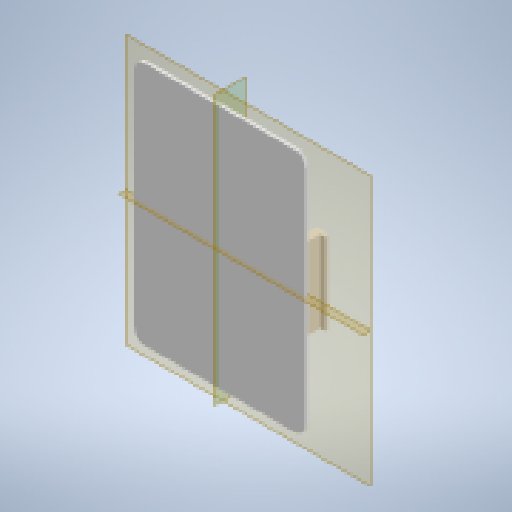
# Autodesk Inventor part: lidV2
Saved by Autodesk Inventor 2025.2 (Build 292293000, 293)
## iProperties
Created: 2022-04-11
Part Number: lidV2
Material: Generic
Document SubType Name: Modeling
Designer: Fred
Density: 1 g/cm^3
Appearance: Default
Author: Fred
Autodesk Inventor part; units mm, degrees
ref_plane "YZ Plane" through (0, 0, 0) normal (1, 0, 0) x (0, 1, 0)
ref_plane "XZ Plane" through (0, 0, 0) normal (0, 1, 0) x (-1, 0, 0)
ref_plane "XY Plane" through (0, 0, 0) normal (0, 0, 1) x (1, 0, 0)
ref_plane "Work Plane1" through (0, 0, 0) normal (0, 0, 1) x (1, 0, 0)
sketch "Sketch1" plane through (0, 0, 0) normal (0, 0, 1) x (1, 0, 0)
  arc A0 (14.605, -35.56) -> (17.78, -32.385) centre (14.605, -32.385) ccw projected
  line L0 (17.78, -32.385) -> (17.78, 33.985) projected
  arc A1 (17.78, 33.985) -> (14.605, 37.16) centre (14.605, 33.985) ccw projected
  line L1 (14.605, 37.16) -> (-29.845, 37.16) projected
  arc A2 (-29.845, 37.16) -> (-33.02, 33.985) centre (-29.845, 33.985) ccw projected
  line L2 (-33.02, 33.985) -> (-33.02, -32.385) projected
  arc A3 (-33.02, -32.385) -> (-29.845, -35.56) centre (-29.845, -32.385) ccw projected
  line L3 (-29.845, -35.56) -> (14.605, -35.56) projected
  line L4 (13.105, -34.06) -> (-28.345, -34.06) projected
  arc A4 (-31.52, -30.885) -> (-28.345, -34.06) centre (-28.345, -30.885) ccw projected
  line L5 (-31.52, -30.885) -> (-31.52, 30.885) projected
  arc A5 (-28.345, 34.06) -> (-31.52, 30.885) centre (-28.345, 30.885) ccw projected
  line L6 (-28.345, 34.06) -> (13.105, 34.06) projected
  arc A6 (16.28, 30.885) -> (13.105, 34.06) centre (13.105, 30.885) ccw projected
  line L7 (16.28, 30.885) -> (16.28, -30.885) projected
  arc A7 (13.105, -34.06) -> (16.28, -30.885) centre (13.105, -30.885) ccw projected
  point P0 (0, 0)
extrude "Extrusion1" add sketch "Sketch1" along normal blind 1 contours L3 A3 L2 A2 L1 A1 L0 A0 | L4 A4 L5 A5 L6 A6 L7 A7
ref_plane "Work Plane2" through (-29.845, 0.8, 0) normal (0, 1, 0) x (1, 0, 0)
sketch "Sketch3" plane through (-29.845, 0.8, 0) normal (0, 1, 0) x (1, 0, 0)
  line L0 (46.125, 31.5) -> (46.125, 0) projected
  line L1 (47.625, 5) -> (47.625, 7) projected
  line L2 (46.125, 5) -> (47.625, 5) projected
  line L3 (46.125, 7) -> (46.125, 5) projected
  line L4 (46.125, 7) -> (47.625, 7) projected
  line L5 (43.375, 0) -> (43.375, 6.8424)
  line L6 (43.375, 6.8424) -> (45.775, 6.8424)
  line L7 (45.775, 6.8424) -> (47.371, 6.0831)
  line L8 (47.371, 6.0831) -> (47.371, 5.3048)
  line L9 (47.371, 5.3048) -> (45.875, 5.3048)
  line L10 (45.875, 5.3048) -> (45.875, 0)
  line L11 (44.45, 0) -> (0, 0) projected
  line L12 (43.375, 0) -> (45.875, 0)
  point P0 (29.845, 0)
  dimension "d17" = 2.5
  dimension "d18" = 0.25
  dimension "d19" = 0.254
  dimension "d20" = 0.3048
  dimension "d21" = 0.1576
  dimension "d23" = 1.496
  dimension "d25" = 115.445
  dimension "d26" = 0.7783
  constraints: 14 end point, 2 perpendicular, 1 collinear, 1 horizontal, 1 parallel, 1 point on line
  measures "d17" distance between parallel lines of L5 L10
  measures "d18" distance between parallel lines of L0 L10
  measures "d19" distance between parallel lines of L1 L8
  measures "d20" distance between parallel lines of L2 L9
  measures "d21" distance between parallel lines of L4 L6
  measures "d23" distance of L8.end L9.end
  measures "d25" angle of L7 L8
  measures "d26" distance of L7.end L8.end
extrude "Extrusion3" add sketch "Sketch3" along normal mid plane 24.13 contours L7 L8 L9 L0 | L0 L9 L10 L12 L11 L5 L6 L7
ref_plane "Work Plane3" through (-7.62, -32.385, 0) normal (-1, 0, 0) x (0, 0, 1)
mirror "Mirror1" about plane through (-7.62, -32.385, 0) normal (-1, 0, 0) of "Extrusion3"
fillet "Fillet1" radius 1.27 1 edges at (13.53, 0.8, 0)
fillet "Fillet2" radius 1.27 1 edges at (-28.77, 0.8, 0)
body "Solid1"
